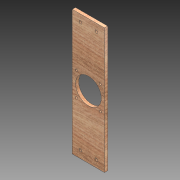
# Autodesk Inventor part: 1223_Motor Plate_V1
Saved by Autodesk Inventor 2020 (Build 240168000, 168)
## iProperties
Created: 2019-09-13
Part Number: 1223_Motor Plate_V1
Material: Wood (Birch)
Document SubType Name: Modeling
Designer: MPI
Density: 0.55 g/cm^3
Appearance: Birch - Natural Polished
Author: MPI
Autodesk Inventor part; units mm, degrees
ref_plane "YZ Plane" through (0, 0, 0) normal (1, 0, 0) x (0, 1, 0)
ref_plane "XZ Plane" through (0, 0, 0) normal (0, 1, 0) x (-1, 0, 0)
ref_plane "XY Plane" through (0, 0, 0) normal (0, 0, 1) x (1, 0, 0)
sketch "Sketch1" plane through (0, 0, 0) normal (0, 1, 0) x (-1, 0, 0)
  line L0 (-50, 195) -> (-50, -195)
  line L1 (50, -195) -> (50, 195)
  circle A0 centre (0, 0) radius 40
  line L2 (70, 37.125) -> (-67, 37.125) construction
  line L3 (70, -37.125) -> (-81, -37.125) construction
  circle A1 centre (37.125, 37.125) radius 3.25
  circle A2 centre (37.125, -37.125) radius 3.25
  circle A3 centre (-37.125, -37.125) radius 3.25
  circle A4 centre (-37.125, 37.125) radius 3.25
  line L4 (50, 195) -> (-50, 195)
  line L5 (50, -195) -> (-50, -195)
  line L6 (97, 172.5) -> (-97, 172.5) construction
  line L7 (88, -172.5) -> (-85, -172.5) construction
  line L8 (-25, 119) -> (-25, -106) construction
  line L9 (25, -106) -> (25, 119) construction
  circle A5 centre (25, 172.5) radius 4.25
  circle A6 centre (-25, 172.5) radius 4.25
  circle A7 centre (-25, -172.5) radius 4.25
  circle A8 centre (25, -172.5) radius 4.25
  dimension "d0" = 80
  dimension "d5" = 74.25
  dimension "d6" = 37.125
  dimension "d7" = 6.5
  dimension "d12" = 74.25
  dimension "d14" = 37.125
  dimension "d15" = 37.125
  dimension "d16" = 37.125
  dimension "d24" = 50
  dimension "d25" = 25
  dimension "d26" = 8.5
  dimension "d29" = 390
  dimension "d30" = 195
  dimension "d31" = 100
  dimension "d32" = 50
  dimension "d33" = 22.5
  dimension "d34" = 22.5
  constraints: 20 end point, 12 point on line, 9 centre point, 6 equal radius, 6 horizontal, 2 parallel, 1 coincident
  measures "d0" diameter of A0
  measures "d5" distance between parallel lines of L3 L2
  measures "d6" distance from line of point (0, 0) L2
  measures "d7" diameter of A1
  measures "d12" distance of A4.centre A1.centre
  measures "d14" horizontal distance of point (0, 0) A4.centre
  measures "d15" horizontal distance of point (0, 0) A3.centre
  measures "d16" horizontal distance of point (0, 0) A2.centre
  measures "d24" distance of L8.end L9.start
  measures "d25" distance from line of point (0, 0) L9
  measures "d26" diameter of A5
  measures "d29" distance of L0.start L0.end
  measures "d30" distance from line of L5 point (0, 0)
  measures "d31" distance of L1.end L0.start
  measures "d32" distance from line of point (0, 0) L1
  measures "d33" distance between parallel lines of L4 L6
  measures "d34" distance between parallel lines of L5 L7
extrude "Extrusion2" add sketch "Sketch1" along normal blind 10
body "Solid2"
